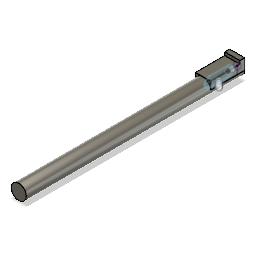
Nintendo 3DS Stylus v4 (Autodesk Fusion 360 design; units mm, degrees)
Autodesk Fusion 360 part; units mm, degrees
sketch "Sketch1" plane through (0, 0, 0) normal (0, 0, 1) x (1, 0, 0)
  circle A0 centre (0, 0) radius 2.45
  dimension "d1" = 4.9
  constraint coincident A0.centre origin
  measures "d1" diameter of A0
extrude "Extrude1" add sketch "Sketch1" along normal blind 70
sketch "Sketch2" plane through (0, 0, 0) normal (0, 0, 1) x (1, 0, 0)
  line L0 (0, 0) -> (2.45, 0)
  line L1 (2.45, 0) -> (-2.45, 0)
  line L2 (-2.45, 0) -> (-2.45, 2.45)
  line L3 (-2.45, 2.45) -> (2.45, 2.45)
  line L4 (2.45, 2.45) -> (2.45, 0)
  dimension "d4" = 2.45
  dimension "d5" = 4.9
  dimension "d6" = 2.45
  constraint coincident L0.start origin
  constraint horizontal L0
  constraint horizontal L1
  constraint vertical L2
  constraint horizontal L3
  constraint vertical L4
  measures "d4" distance of L0.start L0.end
  measures "d5" distance of L0.end L1.end
  measures "d6" distance of L0.end L3.end
extrude "Extrude2" add sketch "Sketch2" along normal blind 11
sketch "Sketch3" plane through (0, 2.45, 0) normal (0, 1, 0) x (-1, 0, 0)
  line L0 (0, 11) -> (-2.45, 11)
  line L1 (-2.45, 11) -> (-2.45, 0)
  line L2 (-2.45, 0) -> (2.45, 0)
  line L3 (2.45, 0) -> (2.45, 11)
  line L4 (2.45, 11) -> (0, 11)
  line L5 (2.45, 0) -> (-2.45, 0)
  line L6 (-2.45, 0) -> (-2.45, 1.6)
  line L7 (-2.45, 1.6) -> (2.45, 1.6)
  line L8 (2.45, 1.6) -> (2.45, 0)
  dimension "d9" = 1.6
  constraint horizontal L5
  constraint vertical L6
  constraint horizontal L7
  constraint vertical L8
  constraint coincident L2.end L3.start
  measures "d9" distance of L2.end L7.end
extrude "Extrude3" add sketch "Sketch3" along normal blind 1 contours L1 L2 L3 L5 L6 L7 L8
sketch "Sketch4" plane through (0, 0, 0) normal (1, 0, 0) x (0, 0, -1)
  line L0 (0, 0) -> (0, -2.45)
  line L1 (0, -2.45) -> (-6.9, -2.45)
  line L2 (-6.9, -2.45) -> (-4.9, -2.45)
  line L3 (-5.9, -2.45) -> (-5.9, -1.825)
  line L4 (-5.9, -1.825) -> (-5.9, -1.325)
  line L5 (-5.9, -1.325) -> (-5.9, -1.2)
  line L6 (0, 0) -> (-0.3154, 0)
  line L7 (-0.3154, 0) -> (-5.9, 0)
  line L8 (-5.9, 0) -> (-2.9, 0)
  line L9 (-5.9, 0) -> (-8.9, 0)
  line L10 (-8.9, 0) -> (-2.9, 0) construction
  line L11 (-1.7, 0) -> (-10.1, 0)
  line L12 (-2.9, 1.575) -> (-8.9, 1.575)
  arc A0 (-8.9, 1.575) -> (-8.9, -1.575) centre (-8.9, 0) ccw
  line L13 (-8.9, -1.575) -> (-2.9, -1.575)
  arc A1 (-2.9, -1.575) -> (-2.9, 1.575) centre (-2.9, 0) ccw
  line L14 (-2.9, 0) -> (-8.9, 0) construction
  line L15 (-10.1, 0) -> (-10.475, 0)
  ellipse E0 centre (-5.9, -2.45) end of major axis (-6.9, -2.45) minor radius 0.5
  line L16 (-4.9, -2.45) -> (-6.9, -2.45) construction
  line L17 (-5.9, -1.95) -> (-5.9, -2.95) construction
  dimension "d12" = 2.45
  dimension "d13" = 6.9
  dimension "d14" = 2
  dimension "d16" = 0.5
  dimension "d17" = 3
  dimension "d18" = 3
  dimension "d29" = 1
  constraint coincident L0.start L6.start
  constraint vertical L0
  constraint perpendicular L0 L1
  constraint parallel L1 L2
  constraint vertical L5
  constraint perpendicular L0 L6
  constraint perpendicular L5 L7
  constraint perpendicular L5 L8
  constraint parallel L8 L9
  constraint coincident L8.end L10.end
  constraint parallel L8 L10
  constraint coincident L9.end L10.start
  constraint tangent L12 A0
  constraint tangent A0 L13
  constraint parallel L12 L13
  constraint tangent L13 A1
  constraint tangent L12 A1
  constraint parallel L10 L14
  constraint midpoint A0 L15.end
  constraint parallel L11 L15
  constraint coincident L2.end E0
  constraint coincident L1.end E0
  measures "d12" distance of L0.start L0.end
  measures "d13" distance of L0.end L1.end
  measures "d14" distance of L1.end L2.end
  measures "d16" distance of L3.end L4.end
  measures "d17" distance of L7.end L8.end
  measures "d18" distance of L7.end L9.end
  measures "d29" distance of E0
extrude "Extrude4" [suppressed]
extrude "Extrude5" [suppressed]
sketch "Sketch5" plane through (0, 0, 70) normal (0, 0, 1) x (1, 0, 0)
  circle A0 centre (0, 0) radius 2.45
  circle A1 centre (0, 0) radius 1.5
  constraint concentric A0 A1
extrude "Extrude6" [suppressed]
fillet "Fillet1" [suppressed]
chamfer "Chamfer1" [suppressed]
moveface "MoveFace1" [suppressed]
fillet "Fillet2" [suppressed]
fillet "Fillet3" [suppressed]
move_face "OffsetFaces1" [suppressed]
moveface "MoveFace2" [suppressed]
sketch "Sketch6" plane through (0, 0, 0) normal (0, 0, 1) x (1, 0, 0)
  circle A0 centre (0, 0) radius 2.45
  line L0 (0, 0) -> (0, -2.45)
  line L1 (0, -2.45) -> (0, -2.95)
  line L2 (0, -2.95) -> (-0.5, -2.95)
  line L3 (-0.5, -2.95) -> (-0.5, -2.3984)
  line L4 (-0.5, -2.3984) -> (0, -2.3984)
  line L5 (0, -2.3984) -> (0, -2.95)
  line L6 (-0.5, -2.95) -> (-0.2, -2.95)
  line L7 (-0.2, -2.95) -> (-1.5058, -1.9327)
  dimension "d30" = 4.9
  dimension "d31" = 0.5
  dimension "d32" = 0.5
  dimension "d33" = 0.3
  constraint coincident A0.centre L0.start
  constraint coincident A0 L0.end
  constraint vertical L0
  constraint parallel L0 L1
  constraint horizontal L2
  constraint vertical L3
  constraint horizontal L4
  constraint vertical L5
  constraint coincident A0 L3.end
  constraint perpendicular L3 L6
  constraint coincident A0 L7.end
  constraint tangent A0 L7
  measures "d30" diameter of A0
  measures "d31" distance of L0.end L1.end
  measures "d32" distance of L1.end L2.end
  measures "d33" distance of L2.end L6.end
move_body "Move2" [suppressed]
equation "d4 = ( 4.9 / 2 ) * 1 mm"
equation "d6 = ( 4.9 / 2 ) * 1 mm"
equation "d12 = ( 4.9 / 2 ) * 1 mm"
equation "d26 = ( 3 / 2 ) * 1 mm"
equation "d28 = ( ( 4.9 - 3 ) / 2 ) * 1 mm"
named bodies: "3DS Stylus"
